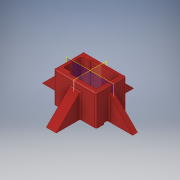
# Autodesk Inventor part: XPivot
Saved by Autodesk Inventor 2017 (Build 210142000, 142)
## iProperties
Created: 2016-11-28
Part Number: XPivot
Material: Generic
Document SubType Name: Modeling
Designer: s4318088
Density: 1 g/cm^3
Appearance: Orange-Red
Author: s4318088
Autodesk Inventor part; units mm, degrees
ref_plane "YZ Plane" through (0, 0, 0) normal (1, 0, 0) x (0, 1, 0)
ref_plane "XZ Plane" through (0, 0, 0) normal (0, 1, 0) x (-1, 0, 0)
ref_plane "XY Plane" through (0, 0, 0) normal (0, 0, 1) x (1, 0, 0)
sketch "Sketch1" plane through (0, 0, 0) normal (0, 1, 0) x (-1, 0, 0)
  line L0 (0, 0) -> (50, 0)
  line L1 (50, 0) -> (50, -32)
  line L2 (50, -32) -> (0, -32)
  line L3 (0, -32) -> (0, 0)
  line L4 (26.15, -5.5) -> (19.5, -5.5)
  line L5 (19.5, -5.5) -> (19.5, -26.5)
  line L6 (19.5, -26.5) -> (26.15, -26.5)
  line L7 (26.15, -26.5) -> (26.15, -5.5)
  dimension "d0" = 50
  dimension "d1" = 32
  dimension "d17" = 6.65
  dimension "d18" = 21
  dimension "d19" = 5.5
  dimension "d20" = 19.5
  constraints: 16 end point, 4 parallel, 2 horizontal, 2 perpendicular
  measures "d0" distance of L1.end L2.end
  measures "d1" distance of L0.end L1.end
  measures "d17" distance of L6.end L5.end
  measures "d18" distance of L5.end L4.end
  measures "d19" distance from line of L2 L6.end
  measures "d20" distance between parallel lines of L3 L5
extrude "Extrusion1" add sketch "Sketch1" along normal blind 10
sketch "Sketch5" plane through (0, 0, 0) normal (0, -1, 0) x (1, 0, 0)
  line L0 (-19.5, -5.5) -> (-26.15, -5.5) projected
  line L1 (-19.5, -5.5) -> (5, -5.5)
  line L2 (5, -26.5) -> (-19.5, -26.5)
  line L3 (-19.5, -26.5) -> (-19.5, -5.5)
  line L4 (-19.5, -26.5) -> (-19.5, -5.5) projected
  line L5 (-19.5, -12.5) -> (5, -12.5)
  line L6 (5, -19.5) -> (-19.5, -19.5)
  line L7 (-19.5, -19.5) -> (-19.5, -12.5)
  line L8 (5, -5.5) -> (5, -12.5)
  line L9 (5, -19.5) -> (5, -26.5)
  dimension "d21" = 21
  dimension "d24" = 7
  dimension "d25" = 7
  dimension "d29" = 24.5
  constraints: 16 end point, 3 point on line, 2 horizontal, 2 parallel
  measures "d21" distance of L1.end L2.start
  measures "d24" distance between parallel lines of L1 L5
  measures "d25" distance between parallel lines of L2 L6
  measures "d29" distance of L0.start L1.end
extrude "Extrusion2" cut sketch "Sketch5" against normal blind 2
sketch "Sketch6" plane through (0, 0, 0) normal (0, -1, 0) x (1, 0, 0)
  line L0 (-19.5, -5.5) -> (-26.15, -5.5) projected
  line L1 (-26.15, -5.5) -> (-26.15, -26.5) projected
  line L2 (-26.15, -26.5) -> (-19.5, -26.5) projected
  line L3 (-19.5, -26.5) -> (-19.5, -5.5) projected
  line L4 (-50, 0) -> (0, 0) projected
  line L5 (0, 0) -> (0, -32) projected
  line L6 (0, -32) -> (-50, -32) projected
  line L7 (-50, -32) -> (-50, 0) projected
  line L8 (-55, 5) -> (5, 5)
  line L9 (5, 5) -> (5, -37)
  line L10 (5, -37) -> (-55, -37)
  line L11 (-55, -37) -> (-55, 5)
  line L12 (-50, -32) -> (-50, 0) projected
  line L13 (-50, -32) -> (0, -32)
  line L14 (0, -32) -> (0, 0)
  line L15 (0, 0) -> (-50, 0)
  line L16 (-50, 0) -> (-50, -32)
  dimension "d26" = 5
  constraints: 16 end point, 2 parallel, 1 horizontal, 1 perpendicular, 3 other
  measures "d26" distance between parallel lines of L7 L11
extrude "Extrusion3" add sketch "Sketch6" against normal blind 43.5 contours L8 L9 L10 L11
sketch "Sketch7" plane through (0, 0, 0) normal (0, -1, 0) x (1, 0, 0)
  line L0 (-55, 5) -> (5, 5) projected
  line L1 (-55, -37) -> (-55, 5) projected
  line L2 (5, -37) -> (-55, -37) projected
  line L3 (5, 5) -> (5, -37) projected
  line L4 (-19.5, -19.5) -> (0, -19.5) projected
  line L5 (0, -19.5) -> (0, -26.5) projected
  line L6 (0, -26.5) -> (-26.15, -26.5) projected
  line L7 (-26.15, -26.5) -> (-26.15, -5.5) projected
  line L8 (-26.15, -5.5) -> (0, -5.5) projected
  line L9 (0, -5.5) -> (0, -12.5) projected
  line L10 (0, -12.5) -> (-19.5, -12.5) projected
  line L11 (-19.5, -12.5) -> (-19.5, -19.5) projected
  line L12 (-19.5, -5.5) -> (0, -5.5) projected
  line L13 (0, -5.5) -> (5, -5.5)
  line L14 (5, -5.5) -> (5, -12.5)
  line L15 (5, -12.5) -> (0, -12.5)
  line L16 (0, -12.5) -> (0, -5.5)
  line L17 (5, 5) -> (5, -37) projected
  line L18 (0, -19.5) -> (5, -19.5)
  line L19 (5, -19.5) -> (5, -26.5)
  line L20 (5, -26.5) -> (0, -26.5)
  line L21 (0, -26.5) -> (0, -19.5)
  point P0 (0, 0)
  constraints: 16 end point, 4 parallel, 2 horizontal, 2 perpendicular, 2 point on line
extrude "Extrusion4" cut sketch "Sketch7" against normal blind 2 contours L3 L15 L9 L13 | L20 L5 L18 L3
fillet "Fillet1" radius 2 8 edges at (-55, 21.75, -37) (-55, 21.75, 5) (5, 21.75, -37) (5, 21.75, 5) (-25, 43.5, -37) (5, 43.5, -16) (-25, 43.5, 5) (-55, 43.5, -16)
sketch "Sketch8" plane through (0, 10, 0) normal (0, 1, 0) x (1, 0, 0)
  line L0 (-19.5, 5.5) -> (-26.15, 5.5) projected
  line L1 (-26.15, 5.5) -> (-26.15, 26.5) projected
  line L2 (-26.15, 26.5) -> (-19.5, 26.5) projected
  line L3 (-19.5, 26.5) -> (-19.5, 5.5) projected
  line L4 (-50, 0) -> (0, 0) projected
  line L5 (0, 0) -> (0, 32) projected
  line L6 (0, 32) -> (-50, 32) projected
  line L7 (-50, 32) -> (-50, 0) projected
  line L8 (-50, 0) -> (0, 0) projected
  line L9 (-50, 0) -> (-38.5, 0)
  line L10 (-38.5, 0) -> (-38.5, 3)
  line L11 (-38.5, 3) -> (-50, 3)
  line L12 (-50, 3) -> (-50, 0)
  line L13 (-50, 32) -> (-38.5, 32)
  line L14 (-38.5, 32) -> (-38.5, 29)
  line L15 (-38.5, 29) -> (-50, 29)
  line L16 (-50, 29) -> (-50, 32)
  dimension "d33" = 11.5
  dimension "d34" = 3
  dimension "d35" = 11.5
  dimension "d36" = 3
  constraints: 16 end point, 4 parallel, 2 horizontal, 2 perpendicular
  measures "d33" distance of L11.end L10.end
  measures "d34" distance of L10.end L9.end
  measures "d35" distance of L14.end L15.end
  measures "d36" distance of L13.end L14.end
extrude "Extrusion5" add sketch "Sketch8" along normal blind 33.5 contours L7 L11 L10 L4 | L7 L6 L14 L15
fillet "Fillet2" radius 2 6 edges at (-38.5, 26.75, 0) (-38.5, 26.75, -3) (-50, 26.75, -3) (-50, 26.75, -29) (-38.5, 26.75, -29) (-38.5, 26.75, -32)
ref_plane "Work Plane1" through (3, 0, -16) normal (0, 0, -1) x (-1, 0, 0)
sketch "Sketch10" plane through (3, 0, -16) normal (0, 0, -1) x (-1, 0, 0)
  line L0 (-2, 41.5) -> (-2, 0) projected
  line L1 (58, 0) -> (58, 41.5) projected
  line L2 (-2, 0) -> (-2, 41.5) projected
  line L3 (-2, 0) -> (-2, 33.5)
  line L4 (-2, 33.5) -> (-35.5, 0)
  line L5 (22.5, 0) -> (-2, 0) projected
  line L6 (-35.5, 0) -> (-2, 0)
  line L7 (0, 0) -> (-2, 0) projected
  line L8 (-2, 33.5) -> (-2, 0)
  line L9 (0, 0) -> (56, 0) projected
  line L10 (28, 0) -> (28, 3.5)
  line L11 (58, 41.5) -> (58, 0)
  line L12 (58, 33.5) -> (91.5, 0)
  line L13 (91.5, 0) -> (58, 0)
  line L14 (58, 0) -> (56, 0) projected
  point P0 (3, 0)
  dimension "d40" = 33.5
  dimension "d41" = 45
  constraints: 16 end point, 2 point on line, 2 symmetric about line, 2 vertical, 1 collinear, 1 midpoint
  measures "d40" distance of L0.end L3.end
  measures "d41" angle of L4 L3
extrude "Extrusion6" add sketch "Sketch10" along normal mid plane 7
fillet "Fillet3" radius 2 6 edges at (-55, 33.5, -16) (-55, 16.75, -19.5) (-55, 16.75, -12.5) (5, 17.75, -12.5) (5, 33.5, -16) (5, 17.75, -19.5)
ref_plane "Work Plane2" through (-25, 0, -26.5) normal (1, 0, 0) x (0, 0, -1)
sketch "Sketch11" plane through (-25, 0, -26.5) normal (1, 0, 0) x (0, 0, -1)
  line L0 (-29.5, 0) -> (-31.5, 0) projected
  line L1 (-31.5, 0) -> (-31.5, 41.5) projected
  line L2 (-31.5, 41.5) -> (-29.5, 41.5) projected
  line L3 (-29.5, 41.5) -> (-29.5, 0) projected
  line L4 (10.5, 41.5) -> (10.5, 0) projected
  line L5 (-31.5, 0) -> (-31.5, 33.5)
  line L6 (-31.5, 0) -> (-31.5, 41.5) projected
  line L7 (-31.5, 33.5) -> (-65, 0)
  line L8 (-65, 0) -> (-31.5, 0)
  line L9 (10.5, 0) -> (10.5, 33.5)
  line L10 (10.5, 33.5) -> (44, 0)
  line L11 (10.5, 0) -> (8.5, 0) projected
  line L12 (44, 0) -> (10.5, 0)
  point P0 (-26.5, 0)
  dimension "d45" = 33.5
  dimension "d46" = 45
  dimension "d47" = 33.5
  dimension "d48" = 45
  constraints: 12 end point, 2 point on line, 1 collinear, 1 perpendicular
  measures "d45" distance of L0.end L5.end
  measures "d46" angle of L7 L5
  measures "d47" distance of L4.end L9.end
  measures "d48" angle of L9 L10
extrude "Extrusion7" add sketch "Sketch11" along normal mid plane 14 contours L8 L7 L1 | L10 L12 L4
fillet "Fillet4" radius 2 6 edges at (-32, 16.75, 5) (-25, 33.5, 5) (-18, 16.75, 5) (-32, 16.75, -37) (-25, 33.5, -37) (-18, 16.75, -37)
sketch "Sketch12" plane through (0, 0, 0) normal (0, -1, 0) x (1, 0, 0)
  point P0 (0, 0)
sketch "Sketch13" plane through (0, 10, 0) normal (0, 1, 0) x (1, 0, 0)
  line L0 (-19.5, 5.5) -> (-26.15, 5.5) projected
  line L1 (-26.15, 5.5) -> (-26.15, 26.5) projected
  line L2 (-26.15, 26.5) -> (-19.5, 26.5) projected
  line L3 (-19.5, 26.5) -> (-19.5, 5.5) projected
  arc A0 (-36.627, 32) -> (-38.5635, 30.5) centre (-36.627, 30) ccw projected
  arc A1 (-40.5, 29) -> (-38.5635, 30.5) centre (-40.5, 31) ccw projected
  line L4 (-40.5, 29) -> (-48, 29) projected
  arc A2 (-48, 29) -> (-50, 27) centre (-48, 27) ccw projected
  line L5 (-50, 27) -> (-50, 5) projected
  arc A3 (-50, 5) -> (-48, 3) centre (-48, 5) ccw projected
  line L6 (-48, 3) -> (-40.373, 3) projected
  arc A4 (-38.4365, 1.5) -> (-40.373, 3) centre (-40.373, 1) ccw projected
  arc A5 (-38.4365, 1.5) -> (-36.5, 0) centre (-36.5, 2) ccw projected
  line L7 (-36.5, 0) -> (0, 0) projected
  line L8 (0, 0) -> (0, 32) projected
  line L9 (0, 32) -> (-36.627, 32) projected
  line L10 (0, 0) -> (0, 32) projected
  line L11 (0, 16) -> (-3.9939, 16)
  point P0 (-2.5, 24)
  point P1 (-2.5, 8)
  point P2 (-8, 2.5)
  point P3 (-16, 2.5)
  point P4 (-24, 2.5)
  point P5 (-32, 2.5)
  point P6 (-8, 29.5)
  point P7 (-16, 29.5)
  point P8 (-24, 29.5)
  point P9 (-32, 29.5)
  dimension "d52" = 2.5
  dimension "d53" = 2.5
  dimension "d54" = 8
  dimension "d55" = 16
  dimension "d56" = 8
  dimension "d57" = 8
  dimension "d58" = 8
  dimension "d59" = 8
  dimension "d60" = 2.5
  dimension "d61" = 2.5
  dimension "d62" = 2.5
  dimension "d63" = 2.5
  constraints: 4 symmetric about line, 2 end point, 1 horizontal, 1 midpoint
  measures "d52" distance from line of L8 point (-2.5, 24)
  measures "d53" distance from line of L8 point (-2.5, 8)
  measures "d54" distance from line of L9 point (-2.5, 24)
  measures "d55" distance of point (-2.5, 24) point (-2.5, 8)
  measures "d56" distance from line of L8 point (-8, 2.5)
  measures "d57" distance of point (-16, 2.5) point (-8, 2.5)
  measures "d58" distance of point (-24, 2.5) point (-16, 2.5)
  measures "d59" distance of point (-32, 2.5) point (-24, 2.5)
  measures "d60" distance from line of L7 point (-32, 2.5)
  measures "d61" distance from line of L7 point (-24, 2.5)
  measures "d62" distance from line of L7 point (-16, 2.5)
  measures "d63" distance from line of L7 point (-8, 2.5)
hole "Hole1" at (-8, 10, -29.5) at (-16, 10, -29.5) at (-24, 10, -29.5) at (-32, 10, -29.5) at (-32, 10, -2.5) at (-24, 10, -2.5) at (-16, 10, -2.5) at (-8, 10, -2.5) at (-2.5, 10, -8) at (-2.5, 10, -24) direction (0, -1, 0) diameter 2 end through all
sketch "Sketch14" plane through (0, 0, 0) normal (0, -1, 0) x (1, 0, 0)
  circle A0 centre (-16, -2.5) radius 1 projected
  circle A1 centre (-32, -2.5) radius 1 projected
  circle A2 centre (-24, -29.5) radius 1 projected
  circle A3 centre (-8, -29.5) radius 1 projected
  circle A4 centre (-16, -29.5) radius 1 projected
  circle A5 centre (-32, -29.5) radius 1 projected
  circle A6 centre (-24, -2.5) radius 1 projected
  circle A7 centre (-8, -2.5) radius 1 projected
  arc A8 (5, 3) -> (3, 5) centre (3, 3) ccw projected
  line L0 (-16, 5) -> (3, 5) projected
  arc A9 (-18, 7) -> (-16, 5) centre (-16, 7) ccw projected
  line L1 (-18, 38.5) -> (-18, 7) projected
  line L2 (-32, 38.5) -> (-18, 38.5) projected
  line L3 (-32, 7) -> (-32, 38.5) projected
  arc A10 (-34, 5) -> (-32, 7) centre (-34, 7) ccw projected
  line L4 (-53, 5) -> (-34, 5) projected
  arc A11 (-53, 5) -> (-55, 3) centre (-53, 3) ccw projected
  line L5 (-55, -10.5) -> (-55, 3) projected
  arc A12 (-57, -12.5) -> (-55, -10.5) centre (-57, -10.5) ccw projected
  line L6 (-88.5, -12.5) -> (-57, -12.5) projected
  line L7 (-88.5, -12.5) -> (-88.5, -19.5) projected
  line L8 (-57, -19.5) -> (-88.5, -19.5) projected
  arc A13 (-55, -21.5) -> (-57, -19.5) centre (-57, -21.5) ccw projected
  line L9 (-55, -35) -> (-55, -21.5) projected
  arc A14 (-55, -35) -> (-53, -37) centre (-53, -35) ccw projected
  line L10 (-34, -37) -> (-53, -37) projected
  arc A15 (-32, -39) -> (-34, -37) centre (-34, -39) ccw projected
  line L11 (-32, -70.5) -> (-32, -39) projected
  line L12 (-32, -70.5) -> (-18, -70.5) projected
  line L13 (-18, -39) -> (-18, -70.5) projected
  arc A16 (-16, -37) -> (-18, -39) centre (-16, -39) ccw projected
  line L14 (3, -37) -> (-16, -37) projected
  arc A17 (3, -37) -> (5, -35) centre (3, -35) ccw projected
  line L15 (5, -26.5) -> (5, -35) projected
  line L16 (5, -26.5) -> (-26.15, -26.5) projected
  line L17 (-26.15, -26.5) -> (-26.15, -5.5) projected
  line L18 (-26.15, -5.5) -> (5, -5.5) projected
  line L19 (5, 3) -> (5, -5.5) projected
  line L20 (-10.1939, -2.5) -> (-9.097, -0.6)
  line L21 (-9.097, -0.6) -> (-6.903, -0.6)
  line L22 (-6.903, -0.6) -> (-5.8061, -2.5)
  line L23 (-5.8061, -2.5) -> (-6.903, -4.4)
  line L24 (-6.903, -4.4) -> (-9.097, -4.4)
  line L25 (-9.097, -4.4) -> (-10.1939, -2.5)
  line L26 (-18.1939, -2.5) -> (-17.097, -0.6)
  line L27 (-17.097, -0.6) -> (-14.903, -0.6)
  line L28 (-14.903, -0.6) -> (-13.8061, -2.5)
  line L29 (-13.8061, -2.5) -> (-14.903, -4.4)
  line L30 (-14.903, -4.4) -> (-17.097, -4.4)
  line L31 (-17.097, -4.4) -> (-18.1939, -2.5)
  line L32 (-26.1939, -2.5) -> (-25.097, -0.6)
  line L33 (-25.097, -0.6) -> (-22.903, -0.6)
  line L34 (-22.903, -0.6) -> (-21.8061, -2.5)
  line L35 (-21.8061, -2.5) -> (-22.903, -4.4)
  line L36 (-22.903, -4.4) -> (-25.097, -4.4)
  line L37 (-25.097, -4.4) -> (-26.1939, -2.5)
  line L38 (-34.1939, -2.5) -> (-33.097, -0.6)
  line L39 (-33.097, -0.6) -> (-30.903, -0.6)
  line L40 (-30.903, -0.6) -> (-29.8061, -2.5)
  line L41 (-29.8061, -2.5) -> (-30.903, -4.4)
  line L42 (-30.903, -4.4) -> (-33.097, -4.4)
  line L43 (-33.097, -4.4) -> (-34.1939, -2.5)
  line L44 (-34.1939, -29.5) -> (-33.097, -27.6)
  line L45 (-33.097, -27.6) -> (-30.903, -27.6)
  line L46 (-30.903, -27.6) -> (-29.8061, -29.5)
  line L47 (-29.8061, -29.5) -> (-30.903, -31.4)
  line L48 (-30.903, -31.4) -> (-33.097, -31.4)
  line L49 (-33.097, -31.4) -> (-34.1939, -29.5)
  line L50 (-26.1939, -29.5) -> (-25.097, -27.6)
  line L51 (-25.097, -27.6) -> (-22.903, -27.6)
  line L52 (-22.903, -27.6) -> (-21.8061, -29.5)
  line L53 (-21.8061, -29.5) -> (-22.903, -31.4)
  line L54 (-22.903, -31.4) -> (-25.097, -31.4)
  line L55 (-25.097, -31.4) -> (-26.1939, -29.5)
  line L56 (-18.1939, -29.5) -> (-17.097, -27.6)
  line L57 (-17.097, -27.6) -> (-14.903, -27.6)
  line L58 (-14.903, -27.6) -> (-13.8061, -29.5)
  line L59 (-13.8061, -29.5) -> (-14.903, -31.4)
  line L60 (-14.903, -31.4) -> (-17.097, -31.4)
  line L61 (-17.097, -31.4) -> (-18.1939, -29.5)
  line L62 (-10.1939, -29.5) -> (-9.097, -27.6)
  line L63 (-9.097, -27.6) -> (-6.903, -27.6)
  line L64 (-6.903, -27.6) -> (-5.8061, -29.5)
  line L65 (-5.8061, -29.5) -> (-6.903, -31.4)
  line L66 (-6.903, -31.4) -> (-9.097, -31.4)
  line L67 (-9.097, -31.4) -> (-10.1939, -29.5)
  point P0 (0, 0)
  dimension "d71" = 1.9
  constraints: 96 end point, 1 coincident, 13 other
  measures "d71" distance from line of A7.centre L24
extrude "Extrusion8" cut sketch "Sketch14" against normal blind 1.7 contours L20 L21 L22 L23 L24 L25 | L26 L27 L28 L29 L30 L31 | L32 L33 L34 L35 L36 L37 | L38 L39 L40 L41 L42 L43 | L44 L45 L46 L47 L48 L49 | L50 L51 L52 L53 L54 L55 | L56 L57 L58 L59 L60 L61 | L62 L63 L64 L65 L66 L67
sketch "Sketch15" plane through (0, 2, 0) normal (0, -1, 0) x (1, 0, 0)
  circle A0 centre (-2.5, -8) radius 1 projected
  line L0 (-19.5, -5.5) -> (5, -5.5) projected
  line L1 (-19.5, -12.5) -> (-19.5, -5.5) projected
  line L2 (7, -12.5) -> (-19.5, -12.5) projected
  arc A1 (5, -10.5) -> (7, -12.5) centre (7, -10.5) ccw projected
  line L3 (5, -5.5) -> (5, -10.5) projected
  circle A2 centre (-2.5, -24) radius 1 projected
  line L4 (-19.5, -19.5) -> (7, -19.5) projected
  line L5 (-19.5, -26.5) -> (-19.5, -19.5) projected
  line L6 (5, -26.5) -> (-19.5, -26.5) projected
  line L7 (5, -21.5) -> (5, -26.5) projected
  arc A3 (7, -19.5) -> (5, -21.5) centre (7, -21.5) ccw projected
  line L8 (-4.6939, -8) -> (-3.597, -6.1)
  line L9 (-3.597, -6.1) -> (-1.403, -6.1)
  line L10 (-1.403, -6.1) -> (-0.3061, -8)
  line L11 (-0.3061, -8) -> (-1.403, -9.9)
  line L12 (-1.403, -9.9) -> (-3.597, -9.9)
  line L13 (-3.597, -9.9) -> (-4.6939, -8)
  line L14 (-4.6939, -24) -> (-3.597, -22.1)
  line L15 (-3.597, -22.1) -> (-1.403, -22.1)
  line L16 (-1.403, -22.1) -> (-0.3061, -24)
  line L17 (-0.3061, -24) -> (-1.403, -25.9)
  line L18 (-1.403, -25.9) -> (-3.597, -25.9)
  line L19 (-3.597, -25.9) -> (-4.6939, -24)
  point P0 (0, 0)
  dimension "d74" = 1.9
  dimension "d75" = 1.9
  constraints: 24 end point, 2 coincident, 26 other
  measures "d74" distance from line of point (-2.5, -8) L12
  measures "d75" distance from line of L15 point (-2.5, -24)
extrude "Extrusion9" cut sketch "Sketch15" against normal blind 1.7 contours L8 L9 L10 L11 L12 L13 | L14 L15 L16 L17 L18 L19
body "Solid1"
